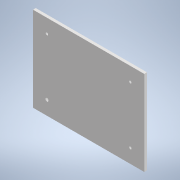
# Autodesk Inventor part: BasePlate
Saved by Autodesk Inventor 2020 (Build 240168000, 168)
## iProperties
Created: 2019-06-17
Part Number: BasePlate
Material: Generic
Document SubType Name: Modeling
Designer: amirt
Density: 1 g/cm^3
Appearance: Default
Author: amirt
Autodesk Inventor part; units mm, degrees
ref_plane "YZ Plane" through (0, 0, 0) normal (1, 0, 0) x (0, 1, 0)
ref_plane "XZ Plane" through (0, 0, 0) normal (0, 1, 0) x (-1, 0, 0)
ref_plane "XY Plane" through (0, 0, 0) normal (0, 0, 1) x (1, 0, 0)
sketch "Sketch1" plane through (0, 0, 0) normal (0, 0, 1) x (1, 0, 0)
  line L0 (12.7, 0) -> (12.7, 12.7)
  circle A0 centre (-76, -52) radius 1.4224 projected
  line L1 (-88.7, -64.7) -> (-76, -64.7)
  line L2 (-88.7, -64.7) -> (12.7, -64.7)
  line L3 (12.7, -64.7) -> (12.7, 12.7)
  line L4 (12.7, 12.7) -> (-88.7, 12.7)
  line L5 (-88.7, 12.7) -> (-88.7, -64.7)
  line L6 (-88.7, 12.7) -> (-76, 12.7)
  line L7 (-88.7, 0) -> (-88.7, 12.7)
  line L8 (-88.7, -64.7) -> (-76, -64.7)
  line L9 (-88.7, -52) -> (-88.7, -64.7)
  line L10 (12.7, -64.7) -> (0, -64.7)
  line L11 (12.7, 12.7) -> (0, 12.7)
  line L12 (12.7, 0) -> (12.7, 12.7)
  circle A1 centre (-76, 0) radius 1.1049
  circle A2 centre (-76, -52) radius 1.1049
  circle A3 centre (0, 0) radius 1.1049
  circle A4 centre (0, -52) radius 1.1049
  dimension "d1" = 12.7
  dimension "d2" = 12.7
  dimension "d10" = 12.7
  dimension "d11" = 12.7
  dimension "d12" = 2.2098
  dimension "d13" = 2.2098
  dimension "d14" = 2.2098
  dimension "d15" = 2.2098
  constraints: 26 end point, 6 coincident, 5 horizontal, 4 centre point, 2 parallel, 1 perpendicular
  measures "d1" distance of L0.end L0.start
  measures "d2" distance of L1.end L1.start
  measures "d10" distance of L12.start point (0, 0)
  measures "d11" distance of point (0, 0) L11.end
  measures "d12" diameter of A1
  measures "d13" diameter of A2
  measures "d14" diameter of A3
  measures "d15" diameter of A4
extrude "Extrusion2" add sketch "Sketch1" against normal blind 2.54 contours L3 L2 L1 L5 L4 L0
body "Solid2"
